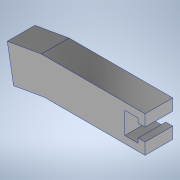
# Autodesk Inventor part: Finray_test_8_Flach_winkel10deg
Saved by Autodesk Inventor 2022 (Build 260153000, 153)
## iProperties
Created: 2022-02-28
Part Number: Finray_test_8_Flach_winkel10deg
Material: Generic
Document SubType Name: Modeling
Designer: richa
Density: 1 g/cm^3
Appearance: Aluminum - Flat
Author: richa
Autodesk Inventor part; units mm, degrees
ref_plane "YZ Plane" through (0, 0, 0) normal (1, 0, 0) x (0, 1, 0)
ref_plane "XZ Plane" through (0, 0, 0) normal (0, 1, 0) x (-1, 0, 0)
ref_plane "XY Plane" through (0, 0, 0) normal (0, 0, 1) x (1, 0, 0)
sketch "Sketch5" plane through (0, 0, 0) normal (0, 0, 1) x (1, 0, 0)
  line L0 (52.8, -15.6) -> (52.8, -10.6)
  line L1 (52.8, -10.6) -> (49.8, -10.6)
  line L2 (49.8, -10.6) -> (49.8, -12.55)
  line L3 (44, -12.55) -> (44, -3.05)
  line L4 (49.8, -3.05) -> (49.8, -5)
  line L5 (49.8, -5) -> (52.8, -5)
  line L6 (52.8, -5) -> (52.8, 0)
  line L7 (52.8, 0) -> (7.8, 0)
  line L8 (44, -3.05) -> (49.8, -3.05)
  line L9 (44, -12.55) -> (49.8, -12.55)
  line L10 (52.8, -15.6) -> (7.8, -15.6)
  arc A0 (7.8, 0) -> (7.8, -15.6) centre (7.8, -7.8) ccw
  point P0 (0, 0)
  dimension "d41" = 5.8
  dimension "d48" = 44
  dimension "d50" = 3
  dimension "d63" = 45
  dimension "d67" = 15.6
  dimension "d71" = 0
  dimension "d72" = 36.2
  dimension "d80" = 5.6
  dimension "d81" = 9.5
  constraints: 22 end point, 7 perpendicular, 4 collinear, 2 parallel, 2 point on circle, 2 tangent, 1 centre point, 1 horizontal, 1 vertical
  measures "d41" distance between parallel lines of L2 L3
  measures "d48" distance from line of L3 point (0, 0)
  measures "d50" distance of L4.end L5.end
  measures "d63" distance of L0.start L10.end
  measures "d67" diameter of A0
  measures "d71" distance from line of point (0, 0) L7
  measures "d72" distance from line of L3 A0.centre
  measures "d80" distance between parallel lines of L5 L1
  measures "d81" distance of L3.start L3.end
extrude "Extrusion2" add sketch "Sketch5" along normal blind 12
sketch "Sketch7" plane through (0, 0, 12) normal (0, 0, 1) x (1, 0, 0)
  line L0 (52.8, 0) -> (7.8, 0) projected
  line L1 (7.8, 0) -> (0, 0)
  line L2 (0, 0) -> (0, -15.6)
  line L3 (0, -15.6) -> (7.8, -15.6)
  line L4 (7.8, -15.6) -> (7.8, 0)
  point P0 (0, 0)
  constraints: 8 end point, 2 parallel, 1 horizontal, 1 perpendicular
extrude "Extrusion4" cut sketch "Sketch7" against normal through all
sketch "Sketch9" plane through (0, 0, 12) normal (0, 0, 1) x (1, 0, 0)
  line L0 (52.8, 0) -> (7.8, 0) projected
  line L1 (7.8, 0) -> (-6.9721, -2.6047)
  line L2 (-6.9721, -2.6047) -> (-4.2632, -17.9677)
  line L3 (-4.2632, -17.9677) -> (10.5089, -15.363)
  line L4 (7.8, 0) -> (10.5089, -15.363)
  line L5 (7.8, 0) -> (7.8, -15.6) projected
  point P0 (0, 0)
  dimension "d83" = 15.6
  dimension "d84" = 10
  dimension "d85" = 90
  dimension "d86" = 10
  dimension "d87" = 15
  constraints: 8 end point, 2 parallel
  measures "d83" distance of L1.end L2.end
  measures "d84" angle of L0 L1
  measures "d85" angle of L2 L3
  measures "d86" angle of L5 L4
  measures "d87" distance of L2.end L3.end
extrude "Extrusion5" add sketch "Sketch9" against normal up to surface (12 mm away)
equation "\"l1\" = 8"
body "Solid2"
